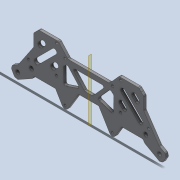
# Autodesk Inventor part: HeadEyeMount
Saved by Autodesk Inventor 2020 (Build 240168000, 168)
## iProperties
Created: 2021-07-13
Part Number: HeadEyeMount
Material: Generic
Document SubType Name: Sheet Metal
Designer: Val
Density: 1 g/cm^3
Sheet Metal Rule: Default
Appearance: Default
Flat Pattern Width: 6.72042 cm
Flat Pattern Length: 18.7942 cm
Flat Pattern Area: 126.305 cm^2
Sheet Metal Width: 2.646 in
Sheet Metal Length: 7.399 in
Sheet Metal Area: 19.577 in^2
Author: Val
Autodesk Inventor part; units mm, degrees
ref_plane "YZ Plane" through (0, 0, 0) normal (1, 0, 0) x (0, 1, 0)
ref_plane "XZ Plane" through (0, 0, 0) normal (0, 1, 0) x (-1, 0, 0)
ref_plane "XY Plane" through (0, 0, 0) normal (0, 0, 1) x (1, 0, 0)
sketch "Base" plane through (0, 0, 0) normal (0, 0, 1) x (1, 0, 0)
  circle A0 centre (69.6753, 73.2321) radius 2.5
  circle A1 centre (86.3368, 60.843) radius 2.5
  line L0 (-0.0001, -227.6975) -> (-0.0001, 252.4162)
  line L1 (85.842, 68.907) -> (66.8769, 97.024)
  line L2 (53.4322, 115.0086) -> (34.2585, 115.0086)
  line L3 (85.842, 68.907) -> (95.5856, 63.4554)
  line L4 (88.9492, 51.5942) -> (68.2683, 63.1652)
  line L5 (68.2683, 63.1652) -> (65.9844, 66.5513)
  line L6 (65.9844, 66.5513) -> (36.1386, 66.5513)
  line L7 (36.1386, 66.5513) -> (12.0154, 74.5903)
  line L8 (95.5856, 63.4554) -> (88.9492, 51.5942)
  line L9 (69.0991, 62.7004) -> (114.921, 37.0627) construction
  line L10 (39.5818, 105.6949) -> (67.736, 63.9544) construction
  line L11 (53.4322, 115.0086) -> (66.8769, 115.0086)
  line L12 (66.8769, 115.0086) -> (66.8769, 97.024)
  line L13 (34.2585, 115.0086) -> (25.3474, 105.0695)
  circle A2 centre (-69.6756, 73.2321) radius 2.5
  circle A3 centre (-86.337, 60.843) radius 2.5
  line L14 (-85.8423, 68.907) -> (-66.8771, 97.024)
  line L15 (-53.4324, 115.0086) -> (-34.2588, 115.0086)
  line L16 (-85.8423, 68.907) -> (-95.5859, 63.4554)
  line L17 (-88.9494, 51.5942) -> (-68.2686, 63.1652)
  line L18 (-68.2686, 63.1652) -> (-65.9847, 66.5513)
  line L19 (-65.9847, 66.5513) -> (-36.1389, 66.5513)
  line L20 (-36.1389, 66.5513) -> (-12.0157, 74.5903)
  line L21 (-95.5859, 63.4554) -> (-88.9494, 51.5942)
  line L22 (-53.4324, 115.0086) -> (-66.8771, 115.0086)
  line L23 (-66.8771, 115.0086) -> (-66.8771, 97.024)
  line L24 (-34.2588, 115.0086) -> (-25.3477, 105.0695)
  line L25 (25.3474, 105.0695) -> (-25.3477, 105.0695)
  line L26 (12.0154, 74.5903) -> (-12.0157, 74.5903)
  circle A4 centre (29.1317, 104.0927) radius 1.38
  circle A5 centre (-28.8683, 104.0927) radius 1.38
  circle A6 centre (-28.8683, 54.8044) radius 1.38
  line L27 (-65.9847, 66.5513) -> (-26.7913, 49.5427)
  line L28 (-26.7913, 49.5427) -> (-24.0411, 55.8802)
  line L29 (-24.0411, 55.8802) -> (-36.1389, 66.5513)
  line L30 (65.9844, 66.5513) -> (26.7911, 49.5427)
  line L31 (26.7911, 49.5427) -> (24.0408, 55.8802)
  line L32 (24.0408, 55.8802) -> (36.1386, 66.5513)
  circle A7 centre (28.8681, 54.8044) radius 1.38
  line L33 (58.8769, 103.4682) -> (55.3364, 107.0086) construction
  line L34 (60.9982, 105.5895) -> (57.4577, 109.1299)
  line L35 (53.2151, 104.8873) -> (56.7555, 101.3468)
  arc A8 (56.7555, 101.3468) -> (60.9982, 105.5895) centre (58.8769, 103.4682) ccw
  arc A9 (57.4577, 109.1299) -> (53.2151, 104.8873) centre (55.3364, 107.0086) ccw
  line L36 (63.2127, 83.576) -> (41.781, 105.0077) construction
  line L37 (61.0913, 81.4547) -> (39.6597, 102.8863)
  line L38 (43.9023, 107.129) -> (65.334, 85.6973)
  arc A10 (61.0913, 81.4547) -> (65.334, 85.6973) centre (63.2127, 83.576) ccw
  arc A11 (43.9023, 107.129) -> (39.6597, 102.8863) centre (41.781, 105.0077) ccw
  line L39 (41.1992, 85.7905) -> (37.6587, 89.3309)
  line L40 (41.9014, 93.5736) -> (45.4418, 90.0331)
  arc A12 (41.1992, 85.7905) -> (45.4418, 90.0331) centre (43.3205, 87.9118) ccw
  arc A13 (41.9014, 93.5736) -> (37.6587, 89.3309) centre (39.7801, 91.4523) ccw
  line L41 (-60.9984, 105.5895) -> (-57.458, 109.1299)
  line L42 (-53.2154, 104.8873) -> (-56.7558, 101.3468)
  arc A14 (-60.9984, 105.5895) -> (-56.7558, 101.3468) centre (-58.8771, 103.4682) ccw
  arc A15 (-53.2154, 104.8873) -> (-57.458, 109.1299) centre (-55.3367, 107.0086) ccw
  line L43 (-61.0916, 81.4547) -> (-39.66, 102.8863)
  line L44 (-43.9026, 107.129) -> (-65.3342, 85.6973)
  arc A16 (-65.3342, 85.6973) -> (-61.0916, 81.4547) centre (-63.2129, 83.576) ccw
  arc A17 (-39.66, 102.8863) -> (-43.9026, 107.129) centre (-41.7813, 105.0077) ccw
  arc A18 (-45.4421, 90.0331) -> (-41.1995, 85.7905) centre (-43.3208, 87.9118) ccw
  line L45 (-41.1995, 85.7905) -> (-37.659, 89.3309)
  line L46 (-41.9017, 93.5736) -> (-45.4421, 90.0331)
  arc A19 (-37.659, 89.3309) -> (-41.9017, 93.5736) centre (-39.7803, 91.4523) ccw
  point P0 (0, 0)
  point P1 (57.1066, 105.2384)
  point P2 (52.4968, 94.2918)
extrude "Plate1" add sketch "Base" along normal blind 3.175 contours L26 L20 L19 L18 L17 L21 L16 L14 L23 L22 L15 L24 L25 L0 | L0 L25 L13 L2 L11 L12 L1 L3 L8 L4 L5 L6 L7 L26
chamfer "BaseChamferFeature" distance 3 angle 45 6 edges at (66.8769, 115.0086, 1.5875) (-66.8771, 115.0086, 1.5875) (95.5856, 63.4554, 1.5875) (88.9492, 51.5942, 1.5875) (-88.9494, 51.5942, 1.5875) (-95.5859, 63.4554, 1.5875)
sketch "CamBottomMountHoles" plane through (0, 0, 3.175) normal (0, 0, 1) x (1, 0, 0)
  circle A0 centre (-38.98, 81.0495) radius 1.05 projected
  circle A1 centre (-73.02, 81.0495) radius 1.05 projected
  point P0 (0, 0)
hole "CamBottomMountHolesFeature" at (-73.02, 81.0495, 3.175) at (-38.98, 81.0495, 3.175) direction (0, 0, -1) diameter 3 end through all
mirror "CamBottomMountHolesMirrorFeature" about plane through (0, 0, 0) normal (1, 0, 0) of "CamBottomMountHolesFeature"
sketch "TopFill" plane through (0, 0, 3.175) normal (0, 0, 1) x (1, 0, 0)
  line L0 (-34.2588, 115.0086) -> (-25.3477, 105.0695)
  line L1 (-34.2588, 115.0086) -> (-36.9485, 118.0086)
  line L2 (-36.9485, 118.0086) -> (-60.8771, 118.0086)
  line L3 (-63.8771, 115.0086) -> (-34.2588, 115.0086)
  line L4 (-60.8771, 118.0086) -> (-63.8771, 115.0086)
  line L5 (-66.8771, 112.0086) -> (-63.8771, 115.0086)
  point P0 (0, 0)
  dimension "d42" = 3
  measures "d42" distance between parallel lines of L2 L3
sheet face with bend "TopFillFeature" sketch "TopFill" thickness 3.175 toward (0, 0, -1) bend radius 3.175 relief straight relief width 3.175 relief depth 1.5875
bend "Bend1"
mirror "TopFillMirrorFeature" about plane through (0, 0, 0) normal (1, 0, 0) of "TopFillFeature"
sketch "Sketch4" plane through (0, 0, 3.175) normal (0, 0, 1) x (1, 0, 0)
  circle A0 centre (-38.98, 115.0895) radius 1.05 projected
  point P0 (0, 0)
hole "EyeMountHolesFeature" at (-38.98, 115.0895, 3.175) direction (0, 0, -1) diameter 3 end through all
mirror "EyeMountHolesMirrorFeatue" about plane through (0, 0, 0) normal (1, 0, 0) of "EyeMountHolesFeature"
sketch "MiddleCut" plane through (0, 0, 3.175) normal (0, 0, 1) x (1, 0, 0)
  line L0 (26.1192, 99.0695) -> (30.5866, 95.0642)
  line L1 (30.5866, 95.0642) -> (30.2682, 74.832)
  line L2 (30.2682, 74.832) -> (10.3422, 81.4723)
  line L3 (36.1386, 66.5513) -> (12.0154, 74.5903) projected
  line L4 (-25.3477, 105.0695) -> (25.3474, 105.0695) projected
  line L5 (34.2588, 115.0086) -> (36.9485, 118.0086) projected
  line L6 (36.1386, 66.5513) -> (36.9485, 118.0086) construction
  line L7 (25.3474, 105.0695) -> (34.2585, 115.0086) projected
  line L8 (-12.0157, 74.5903) -> (12.0154, 74.5903) projected
  line L9 (-0.0001, 74.5903) -> (-0.0001, 105.0695) construction
  line L10 (-26.1195, 99.0695) -> (-30.5869, 95.0642)
  line L11 (-30.5869, 95.0642) -> (-30.2685, 74.832)
  line L12 (-30.2685, 74.832) -> (-10.3424, 81.4723)
  line L13 (-26.1195, 99.0695) -> (26.1192, 99.0695)
  line L14 (-10.3424, 81.4723) -> (10.3422, 81.4723)
  line L15 (-26.1195, 99.0695) -> (-10.3424, 81.4723)
  line L16 (10.3422, 81.4723) -> (26.1192, 99.0695)
  line L17 (-20.7472, 99.0695) -> (-4.9702, 81.4723)
  line L18 (4.9699, 81.4723) -> (20.747, 99.0695)
  point P0 (0, 0)
  dimension "d56" = 6
  dimension "d57" = 6
  dimension "d58" = 6
  dimension "d63" = 6
  dimension "d64" = 4
  dimension "d65" = 4
  constraints: 28 end point, 5 parallel, 4 point on line, 4 symmetric about line, 2 midpoint, 2 perpendicular, 1 horizontal
  measures "d56" distance between parallel lines of L3 L2
  measures "d57" distance between parallel lines of L6 L1
  measures "d58" distance of L0.start L0.end
  measures "d63" distance between parallel lines of L4 L13
  measures "d64" distance between parallel lines of L17 L15
  measures "d65" distance between parallel lines of L16 L18
extrude "MiddleCutFeature" cut sketch "MiddleCut" against normal blind 3.175 contours L0 L1 L2 L16 | L18 L14 L17 L13 | L15 L12 L11 L10
fillet "FilletsFeature" radius 2 40 edges at (-26.1195, 99.0695, 1.5875) (-30.5869, 95.0642, 1.5875) (-30.2685, 74.832, 1.5875) (-10.3424, 81.4723, 1.5875) (20.747, 99.0695, 1.5875) (-20.7472, 99.0695, 1.5875) (4.9699, 81.4723, 1.5875) (-4.9702, 81.4723, 1.5875) (10.3422, 81.4723, 1.5875) (30.2682, 74.832, 1.5875) (30.5866, 95.0642, 1.5875) (26.1192, 99.0695, 1.5875) (-25.3477, 105.0695, 1.5875) (-36.9485, 118.0086, 1.5875) (-60.8771, 118.0086, 1.5875) (-66.8771, 112.0086, 1.5875) (-66.8771, 97.024, 1.5875) (-85.8423, 68.907, 1.5875) (-92.9678, 64.9202, 1.5875) (-94.121, 60.8373, 1.5875) (-90.4143, 54.2122, 1.5875) (-86.3314, 53.059, 1.5875) (-68.2686, 63.1652, 1.5875) (-65.9847, 66.5513, 1.5875) (-36.1389, 66.5513, 1.5875) (-12.0157, 74.5903, 1.5875) (12.0154, 74.5903, 1.5875) (36.1386, 66.5513, 1.5875) (65.9844, 66.5513, 1.5875) (68.2683, 63.1652, 1.5875) (86.3311, 53.059, 1.5875) (90.414, 54.2122, 1.5875) (94.1208, 60.8373, 1.5875) (92.9675, 64.9202, 1.5875) (85.842, 68.907, 1.5875) (66.8769, 97.024, 1.5875) (66.8769, 112.0086, 1.5875) (60.8771, 118.0086, 1.5875) (36.9485, 118.0086, 1.5875) (25.3474, 105.0695, 1.5875)
sketch "Sketch6" plane through (0, 0, 0) normal (0, 0, -1) x (-1, 0, 0)
  circle A0 centre (28.8683, 54.8044) radius 1.2295
  line L0 (30.1161, 56.6767) -> (31.1137, 54.6599)
  line L1 (31.1137, 54.6599) -> (29.8659, 52.7876)
  circle A1 centre (28.8683, 54.8044) radius 4
  line L2 (28.8683, 54.8044) -> (35.8311, 66.6539) construction
  line L3 (12.3235, 74.4877) -> (35.8311, 66.6539) construction
  line L4 (25.4432, 52.7383) -> (12.3235, 74.4877)
  line L5 (32.317, 52.778) -> (40.4102, 66.5513)
  line L6 (36.4634, 66.5513) -> (64.9213, 66.5513) construction
  line L7 (12.3235, 74.4877) -> (35.8311, 66.6539)
  line L8 (35.8311, 66.6539) -> (40.4102, 66.5513)
  point P0 (0, 0)
  dimension "d67" = 8
  measures "d67" diameter of A1
sheet face with bend "Face3" sketch "Sketch6" thickness 3.175 toward (0, 0, 1) bend radius 3.175 relief straight relief width 3.175 relief depth 1.5875
bend "Bend2"
ref_plane "Work Plane1" through (-0.0001, 69.9368, 3.175) normal (1, 0, 0) x (0, 0, 1)
mirror "Mirror4" about plane through (-0.0001, 69.9368, 3.175) normal (1, 0, 0) of "Face3"
ref_plane "Work Plane2" through (-0.0001, 69.9368, 3.175) normal (1, 0, 0) x (0, 0, 1)
equation "\"d61\" = Thickness"
equation "\"d9\" = Thickness"
equation "\"d43\" = BendRadius"
equation "\"d44\" = BendReliefWidth"
equation "\"d46\" = MinimumRemnant"
equation "\"d45\" = BendReliefDepth"
equation "\"d47\" = TransitionRadius"
equation "\"BendRadius\" = Thickness"
equation "\"BendReliefWidth\" = Thickness"
equation "\"BendReliefDepth\" = 0.5 * Thickness"
equation "\"CornerReliefSize\" = 4 * Thickness"
equation "\"MinimumRemnant\" = 2 * Thickness"
equation "\"TransitionRadius\" = BendRadius"
equation "\"JacobiRadiusSize\" = BendRadius"
equation "\"GapSize\" = Thickness"
equation "\"d1\" = d0"
equation "\"d2\" = d0"
equation "\"Thickness\" = 3.175"
equation "\"d0\" = 6.795788"
body "Solid1"
